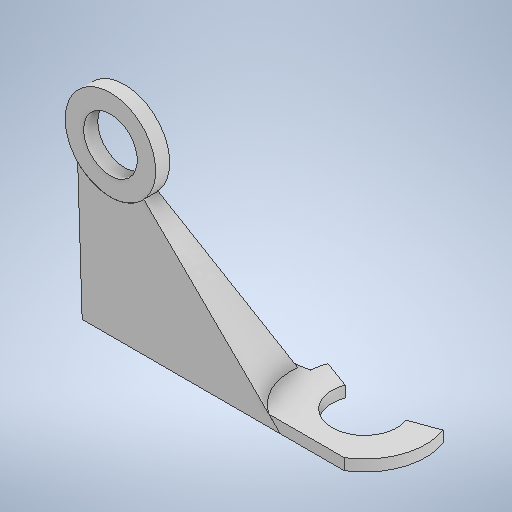
# Autodesk Inventor part: Pot_mount_best
Saved by Autodesk Inventor 2025.1 (Build 291241000, 241)
## iProperties
Created: 2025-05-22
Part Number: Pot_mount_best
Material: Generic
Document SubType Name: Modeling
Designer: Andreas' PC
Density: 1 g/cm^3
Appearance: Default
Author: Andreas' PC
Autodesk Inventor part; units mm, degrees
ref_plane "Work Plane6" through (14.4702, 32.0662, 39.5) normal (0, 0, 1) x (1, 0, 0)
sketch "Sketch1" plane through (14.4702, 32.0662, 39.5) normal (0, 0, 1) x (1, 0, 0)
  point P0 (-14.4702, -32.0662)
ref_plane "Work Plane1" through (14.4702, 32.0662, 47.5) normal (0, 0, -1) x (-1, 0.0032, 0)
sketch "Sketch2" plane through (14.4702, 32.0662, 47.5) normal (0, 0, -1) x (-1, 0.0032, 0)
  line L0 (-3.06, 5.3) -> (3.06, 5.3)
  line L1 (3.06, 5.3) -> (6.1199, 0)
  line L2 (6.1199, 0) -> (3.06, -5.3)
  line L3 (3.06, -5.3) -> (-3.06, -5.3)
  line L4 (-3.06, -5.3) -> (-6.1199, 0)
  line L5 (-6.1199, 0) -> (-3.06, 5.3)
  circle A0 centre (0, 0) radius 8
  line L6 (-3.06, -5.3) -> (-3.06, 5.3)
  line L7 (-3.06, 5.3) -> (-8, 5.3)
  line L8 (-8, 5.3) -> (-8, -5.3)
  line L9 (-8, -5.3) -> (-3.06, -5.3)
  circle A1 centre (0, 0) radius 4.75
  point P0 (14.3663, -32.1129)
  point P1 (-5.9925, -5.3)
  point P2 (-5.9925, 5.3)
  point P3 (-3.06, 3.6331)
  point P4 (-3.06, -3.6331)
  point P5 (-3.06, -5.3)
  point P6 (-3.06, 5.3)
  point P7 (-3.06, -5.3)
  point P8 (-3.06, 5.3)
  point P9 (-3.06, -5.3)
  point P10 (-8, 0)
  point P11 (-3.06, 5.3)
  point P12 (-3.06, -5.3)
  dimension "d3" = 10.6
  dimension "d4" = 16
  dimension "d9" = 9.5
  constraints: 20 end point, 2 centre point, 2 coincident, 2 parallel, 1 perpendicular, 1 other
  measures "d3" distance between parallel lines of L3 L0
  measures "d4" diameter of A0
  measures "d9" diameter of A1
extrude "Extrusion1" add sketch "Sketch2" against normal blind 2.5 contours L7 A0 L9 L3 L2 L1 L0 | L6 A1 L4 L5 | L0 L1 L2 L3 L6 A1 | L5 L4 L9 A0 L7
ref_plane "Work Plane2" through (14.4702, 32.0662, 46.35) normal (0, 0, -1) x (-1, 0.0032, 0)
ref_plane "Work Plane4" through (20.4455, 26.7469, 47.5) normal (0.0032, 1, 0) x (1, -0.0032, 0)
sketch "Sketch5" plane through (20.4455, 26.7469, 47.5) normal (0.0032, 1, 0) x (1, -0.0032, 0)
  line L0 (-13.9925, -2.5) -> (2.0075, -2.5) projected
  line L1 (2.0075, 0) -> (-13.9925, 0) projected
  line L2 (-0.1528, -2.5) -> (-0.1528, 0)
  line L3 (-11.7789, -2.5) -> (-11.7789, 0)
  line L4 (2.0075, 0) -> (-13.9925, 0) projected
  point P0 (-20.3588, 47.5)
  constraints: 4 end point, 4 point on line, 1 parallel, 1 perpendicular
ref_plane "Work Plane7" through (-59.5298, 2.0662, -55) normal (0, 1, 0) x (1, 0, 0)
sketch "Sketch6" plane through (-59.5298, 2.0662, -55) normal (0, 1, 0) x (1, 0, 0)
  circle A0 centre (109, -95) radius 5.35 projected
  circle A1 centre (109, -95) radius 5.75
  circle A2 centre (109, -95) radius 10.8507
  line L0 (109, -95) -> (98.8037, -91.2888)
  line L1 (109, -95) -> (119.1963, -91.2888)
  line L2 (109, -95) -> (98.1493, -95)
  line L3 (66.0434, -104.5) -> (82.0433, -104.5) projected
  line L4 (82.0433, -104.5) -> (114.2428, -104.5)
  line L5 (66, -105) -> (82, -105) projected
  line L6 (66, -104.5) -> (82, -104.5) projected
  line L7 (82, -105.5) -> (82.0433, -105.5) projected
  point P0 (59.5298, -55)
  point P1 (103.5968, -93.0334)
  point P2 (114.4032, -93.0334)
  point P3 (103.7572, -104.5)
  dimension "d12" = 11.5
  dimension "d13" = 20
  dimension "d14" = 160
  constraints: 8 end point, 4 point on circle, 2 centre point, 2 coincident, 1 horizontal
  measures "d12" diameter of A1
  measures "d13" angle of L0 L2
  measures "d14" angle of L2 L1
extrude "Extrusion3" add sketch "Sketch6" along normal blind 2 contours L1 A2 L4 L2 A1 | L2 A2 L0 A1
ref_plane "Work Plane8" through (-59.5298, 2.0662, -55) normal (0, 1, 0) x (1, 0, 0)
sketch "Sketch7" plane through (-59.5298, 2.0662, -55) normal (0, 1, 0) x (1, 0, 0)
  line L0 (68.2541, -98.4179) -> (68.2541, -104.2594) projected
  line L1 (79.6782, -98.4179) -> (79.6782, -104.2594) construction
  line L2 (68.2541, -98.4179) -> (103.5968, -93.0334)
  line L3 (68.2541, -104.2594) -> (103.343, -104.2594)
  arc A0 (98.8037, -91.2888) -> (119.1963, -91.2888) centre (109, -95) ccw projected
  line L4 (103.5968, -93.0334) -> (98.8037, -91.2888) projected
  arc A1 (103.5968, -93.0334) -> (109, -100.75) centre (109, -95) ccw
  line L5 (103.343, -104.2594) -> (109, -100.75)
  arc A2 (98.21, -93.8541) -> (103.343, -104.2594) centre (109, -95) ccw
  line L6 (103.343, -104.2594) -> (114.657, -104.2594)
  circle A3 centre (109, -95) radius 10.8507 projected
  point P0 (59.5298, -55)
  constraints: 8 end point, 7 point on circle, 2 centre point, 2 horizontal, 1 concentric, 1 point on line
loft "Loft1" add profiles "Sketch7", "Sketch5" contours L2 A0 L3 L0 / all
extrude "Extrusion4" add sketch "Sketch7" along normal blind 2 contours L2 A0 L3 L0
ref_plane "Work Plane5" through (-59.5298, 2.0662, -55) normal (0, 1, 0) x (1, 0, 0)
sketch "Sketch9" plane through (-59.5298, 2.0662, -55) normal (0, 1, 0) x (1, 0, 0)
  point P0 (59.5298, -55)
extrude "Extrusion6" cut sketch "Sketch7" along normal blind 10 contours L6 A0
body "Solid1"
